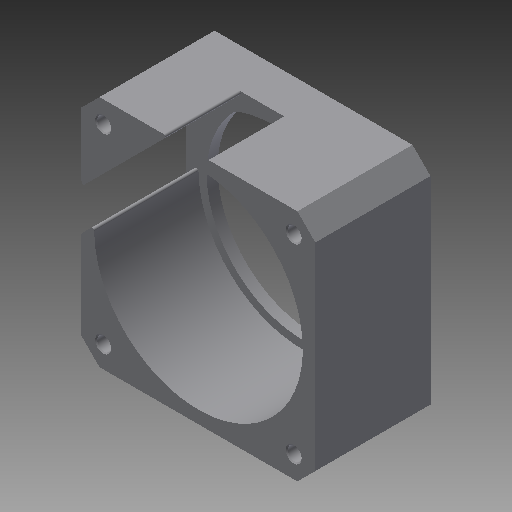
# Autodesk Inventor part: Корпус
Saved by Autodesk Inventor 2022 (Build 260153000, 153)
## iProperties
RuleStatus: InUse
Part Number: Корпус
Checked By: Якушев
Engr Approved By: Малов
Material: По умолчанию1
Document SubType Name: Modeling
Mfg Approved By: Судаков
Designer: Смирнов
Density: 1 g/cm^3
Appearance: По умолчанию1
Mass: 45.9951 g
Surface Area: 182.84 cm^2
Volume: 45.9951 cm^3
AfterMaterialChange0: Материал
BeforeDocSave0: Материал
AfterAnyiPropertyChange0: Материал
Материал: По умолчанию1
Author: Смирнов
Title: Корпус
Autodesk Inventor part; units mm, degrees
ref_plane "РабПлоскость1" through (0, 0, 43.2) normal (0, 0, 1) x (1, 0, 0)
sketch "Эскиз1" plane through (0, 0, 43.2) normal (0, 0, 1) x (1, 0, 0)
  circle A0 centre (0, 0) radius 12.5 construction
  circle A1 centre (26.4645, -26.4645) radius 1.95 construction
  circle A2 centre (-26.4645, 26.4645) radius 1.95 construction
  circle A3 centre (26.4645, 26.4645) radius 1.95 construction
  circle A4 centre (-26.4645, -26.4645) radius 1.95 construction
  circle A5 centre (15.35, -15.35) radius 3.3 construction
  circle A6 centre (-15.35, 15.35) radius 3.3 construction
  circle A7 centre (15.35, 15.35) radius 3.3 construction
  circle A8 centre (-15.35, -15.35) radius 3.3 construction
  line L0 (-32.5, 27.5) -> (-32.5, -27.5) projected
  line L1 (-32.5, -27.5) -> (-27.5, -32.5) projected
  line L2 (-27.5, -32.5) -> (27.5, -32.5) projected
  line L3 (27.5, -32.5) -> (32.5, -27.5) projected
  line L4 (32.5, -27.5) -> (32.5, 27.5) projected
  line L5 (32.5, 27.5) -> (27.5, 32.5) projected
  line L6 (27.5, 32.5) -> (-27.5, 32.5) projected
  line L7 (-27.5, 32.5) -> (-32.5, 27.5) projected
  circle A9 centre (-26.4645, 26.4645) radius 1.7
  circle A10 centre (-26.4645, -26.4645) radius 1.7
  circle A11 centre (26.4645, -26.4645) radius 1.7
  circle A12 centre (26.4645, 26.4645) radius 1.7
  point P0 (0, 0)
  dimension "d0" = 3.4
  dimension "d3" = 360
  constraints: 4 centre point, 1 coincident, 9 other
  measures "d0" diameter of A9
ref_plane "РабПлоскость2" through (-24, -24, 68.2) normal (0, 0, 1) x (1, 0, 0)
ref_plane "РабПлоскость3" through (-25, -25, 76.2) normal (0, 0, 1) x (1, 0, 0)
ref_plane "РабПлоскость4" through (-25, -25, 75.2) normal (0, 0, 1) x (1, 0, 0)
extrude "Выдавливание1" add sketch "Эскиз1" along normal up to surface (32 mm away)
sketch "Эскиз2" plane through (-27.5, -32.5, 75.2) normal (0, 0, 1) x (1, 0, 0)
  circle A0 centre (27.5, 32.5) radius 26.7
  circle A1 centre (27.5, 32.5) radius 26 construction
  point P0 (27.5, 32.5)
  dimension "d7" = 0.7
  constraints: 1 centre point, 1 coincident
  measures "d7" radial gap between concentric circles of A0 A1
extrude "Выдавливание2" cut sketch "Эскиз2" against normal through all
sketch "Эскиз3" plane through (-27.5, -32.5, 75.2) normal (0, 0, 1) x (1, 0, 0)
  circle A0 centre (27.5, 32.5) radius 29
  point P0 (27.5, 32.5)
  dimension "d10" = 58
  constraints: 1 centre point, 1 coincident
  measures "d10" diameter of A0
extrude "Выдавливание3" cut sketch "Эскиз3" against normal blind 29
sketch "Эскиз4" plane through (-27.5, -32.5, 75.2) normal (0, 0, 1) x (1, 0, 0)
  line L0 (27.5, 32.5) -> (-17.4216, 32.5) construction
  line L1 (27.5, 32.5) -> (27.5, 86.8175) construction
  line L2 (-5, 5) -> (-5, 60) construction
  line L3 (30.3015, 65) -> (-5, 29.6985)
  line L4 (-5, 29.6985) -> (-10.6569, 35.3553)
  line L5 (-10.6569, 35.3553) -> (24.6447, 70.6569)
  line L6 (24.6447, 70.6569) -> (30.3015, 65)
  line L7 (30.3015, 65) -> (-10.6569, 35.3553) construction
  line L8 (-5, 29.6985) -> (24.6447, 70.6569) construction
  line L9 (-5, 60) -> (0, 65) construction
  line L10 (0, 65) -> (55, 65) construction
  circle A0 centre (27.5, 32.5) radius 29 construction
  point P0 (9.8223, 50.1777)
  dimension "d16" = 8
  constraints: 16 end point, 3 parallel, 2 midpoint, 2 point on line, 1 horizontal, 1 perpendicular, 1 tangent, 1 vertical
  measures "d16" distance of L5.end L3.start
extrude "Выдавливание4" cut sketch "Эскиз4" against normal up to surface (29 mm away)
sketch "Эскиз5" plane through (-27.5, -32.5, 46.2) normal (0, 0, 1) x (1, 0, 0)
  arc A0 (-1.4914, 33.2071) -> (26.7929, 61.4914) centre (27.5, 32.5) ccw projected
  line L0 (30.3015, 65) -> (26.7929, 61.4914) projected
  line L1 (18.9878, 65) -> (30.3015, 65) projected
  line L2 (-5, 41.0122) -> (18.9878, 65) projected
  line L3 (-5, 29.6985) -> (-5, 41.0122) projected
  line L4 (-1.4914, 33.2071) -> (-5, 29.6985) projected
  circle A1 centre (27.5, 32.5) radius 26.7 projected
  circle A2 centre (27.5, 32.5) radius 29
  point P0 (27.5, 32.5)
  point P1 (6.9939, 53.0061)
  constraints: 1 coincident, 3 other
extrude "Выдавливание5" add sketch "Эскиз5" along normal blind 8 contours L2 L1 L0 A2
fillet "Сопряжение1" radius 0.5 6 edges at (-0.7071, 28.9914, 64.7) (-28.9914, 0.7071, 60.7) (-8.5122, 32.5, 64.7) (2.8015, 32.5, 64.7) (-32.5, -2.8015, 60.7) (-32.5, 8.5122, 60.7)
sketch "Эскиз6" plane through (-27.5, -32.5, 75.2) normal (0, 0, 1) x (1, 0, 0)
  circle A0 centre (1.0355, 58.9645) radius 1.7 construction
  circle A1 centre (53.9645, 58.9645) radius 1.7 construction
  circle A2 centre (53.9645, 6.0355) radius 1.7 construction
  circle A3 centre (1.0355, 6.0355) radius 1.7 construction
  point P0 (27.5, 32.5)
hole "Отверстие1" at (-26.4645, 26.4645, 75.2) at (26.4645, 26.4645, 75.2) at (26.4645, -26.4645, 75.2) at (-26.4645, -26.4645, 75.2) direction (0, 0, -1) diameter 3.9 depth 8 countersink diameter 4.5 countersink angle 90
ref_plane "РабПлоскость5" through (-27.5, -32.5, 59.2) normal (0, 0, 1) x (1, 0, 0)
mirror "Зеркальное отражение1" about plane through (-27.5, -32.5, 59.2) normal (0, 0, 1) of "Отверстие1"
